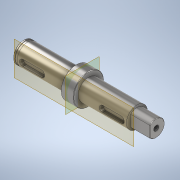
# Autodesk Inventor part: ParallelSystem_ProximalPart_Shaft_Driven_Rillenkugellager
Saved by Autodesk Inventor 2022 (Build 260153000, 153)
## iProperties
Created: 2022-07-19
Part Number: ParallelSystem_ProximalPart_Shaft_Driven_Rillenkugellager
Material: Edelstahl
Document SubType Name: Modeling
Designer: alexw
Density: 8 g/cm^3
Appearance: Halbpoliert
Mass: 39.624 g
Surface Area: 24.2962 cm^2
Volume: 4.95301 cm^3
ParrallelMecha_DrivenLink_OuterWidth: 52,000 mm
Querstrebe_Length: 36,000 mm
Author: alexw
Autodesk Inventor part; units mm, degrees
ref_plane "YZ Plane" through (0, 0, 0) normal (1, 0, 0) x (0, 1, 0)
ref_plane "XZ Plane" through (0, 0, 0) normal (0, 1, 0) x (-1, 0, 0)
sketch "Skizze1" plane through (0, 0, 0) normal (0, 0, 1) x (1, 0, 0)
  line L0 (0, 0) -> (0, 5)
  line L1 (0, 5) -> (0.8, 5)
  line L2 (0.8, 5) -> (0.8, 4.8)
  line L3 (0.8, 4.8) -> (1.9, 4.8)
  line L4 (1.9, 4.8) -> (1.9, 5)
  line L5 (1.9, 5) -> (24.9, 5)
  line L6 (24.9, 5) -> (24.9, 7.25)
  line L7 (24.9, 7.25) -> (30.9, 7.25)
  line L8 (30.9, 7.25) -> (30.9, 5)
  line L9 (30.9, 5) -> (53.9, 5)
  line L10 (53.9, 5) -> (53.9, 4)
  line L11 (53.9, 4) -> (63.1, 4)
  line L12 (63.1, 4) -> (63.1, 0)
  line L13 (63.1, 0) -> (0, 0)
  line L14 (15.9, 5) -> (15.9, 0) construction
  line L15 (39.9, 5) -> (39.9, 0) construction
  line L16 (9.9, 5) -> (9.9, 0) construction
  line L17 (45.9, 5) -> (45.9, 0) construction
  line L18 (53.9, 5) -> (53.9, 0) construction
  dimension "d0" = 10
  dimension "d2" = 14.5
  dimension "d3" = 1.1
  dimension "d4" = 9.6
  dimension "d5" = 0.8
  dimension "d7" = 9
  dimension "d8" = 9
  dimension "d9" = 6
  dimension "d10" = 14
  dimension "d11" = 14
  dimension "ParrallelMecha_DrivenLink_OuterWidth" = 52
  dimension "d22" = 6
  dimension "d23" = 6
  dimension "Querstrebe_Length" = 36
  dimension "d25" = 9.2
  dimension "d26" = 8
  constraints: 38 end point, 14 perpendicular, 13 point on line, 1 vertical
  measures "d0" diameter of L5 L13
  measures "d2" diameter of L7 L13
  measures "d3" distance of L3.end L2.end
  measures "d4" diameter of L3 L13
  measures "d5" distance between parallel lines of L2 L0
  measures "d7" distance between parallel lines of L6 L14
  measures "d8" distance between parallel lines of L8 L15
  measures "d9" distance between parallel lines of L8 L6
  measures "d10" distance between parallel lines of L4 L14
  measures "d11" distance between parallel lines of L15 L10
  measures "ParrallelMecha_DrivenLink_OuterWidth" distance between parallel lines of L10 L4
  measures "d22" distance between parallel lines of L15 L17
  measures "d23" distance between parallel lines of L16 L14
  measures "Querstrebe_Length" distance between parallel lines of L17 L16
  measures "d25" distance between parallel lines of L12 L18
  measures "d26" diameter of L11 L13
revolve "Umdrehung1" add sketch "Skizze1" angle 360 about axis through (63.1, 0, 0) along (-1, 0, 0)
chamfer "Fase1" distance 0.2 angle 45 4 edges at (24.9, -7.25, 0) (30.9, -7.25, 0) (63.1, -4, 0) (0, -5, 0)
ref_plane "Wellennut_Spiegelebene" through (27.9, 0, 0) normal (-1, 0, 0) x (0, 0, 1)
ref_plane "Arbeitsebene2" through (13.4, 0, 5) normal (0, 0, 1) x (1, 0, 0)
sketch "Skizze3" plane through (13.4, 0, 5) normal (0, 0, 1) x (1, 0, 0)
  line L0 (2.5, 5) -> (2.5, 0) construction
  line L1 (-26.02, 0) -> (62.32, 0) construction
  line L2 (0, 0) -> (-9, 0) construction
  line L3 (0, 1.5) -> (-9, 1.5)
  line L4 (-9, -1.5) -> (0, -1.5)
  arc A0 (0, -1.5) -> (0, 1.5) centre (0, 0) ccw
  arc A1 (-9, 1.5) -> (-9, -1.5) centre (-9, 0) ccw
  line L5 (-11.5, 0) -> (2.5, 0) construction
  line L6 (-11.5, -5) -> (-11.5, 5) construction
  point P0 (-13.4, 0)
  point P1 (-4.5, 0)
  point P2 (-4.5, 0)
  dimension "d17" = 3
  dimension "d18" = 12
  constraints: 10 end point, 4 point on circle, 4 tangent, 3 midpoint, 2 centre point, 2 horizontal, 2 point on line, 1 coincident, 1 collinear, 1 parallel
  measures "d17" distance between parallel lines of L4 L3
extrude "Wellennut" cut sketch "Skizze3" against normal blind 1.8
mirror "Spiegeln1" about plane through (27.9, 0, 0) normal (-1, 0, 0) of "Wellennut"
sketch "Skizze4" plane through (53.9, 0, 0) normal (1, 0, 0) x (0, 0, -1)
  circle A0 centre (0, 0) radius 4 projected
  line L0 (-3, -2.6458) -> (-3, 2.6458)
  point P0 (0, 0)
  dimension "d27" = 3
  constraints: 2 end point, 2 point on circle, 1 vertical
  measures "d27" distance from line of L0 point (0, 0)
extrude "Extrusion2" cut sketch "Skizze4" along normal through all contours L0 A0 picked at (-3.1815, -0.6179)
chamfer "Fase2" distance 0.2 angle 45 1 edges at (63.1, 0, 3)
sketch "Skizze5" plane through (63.1, 0, 0) normal (1, 0, 0) x (0, 0, -1)
  arc A0 (-3, -2.6458) -> (-3, 2.6458) centre (0, 0) ccw construction
  circle A1 centre (0, 0) radius 5 construction
  point P0 (0, 0)
  constraints: 1 coincident
hole "Bohrung1" at (63.1, 0, 0) direction (-1, 0, 0) diameter 2.459 depth 8 tip angle 118 thread size "M3x0.5" class "6H" standard "ISO Metric profile"
equation "\"d10\" = ParallelLink_Lever_Thickness + ParallelMecha_Bearing_Step_Thickness"
equation "\"d11\" = d10"
equation "\"d22\" = ParallelMecha_Bearing_Step_Thickness"
equation "\"d23\" = d22"
equation "\"d26\" = CapstonV2_ShaftDia"
equation "\"d27\" = 0.5 * CapstonV2_ShaftDia - Poligonprofil_Ausnehmung"
equation "\"ParallelLink_Lever_Thickness\" = 8"
equation "\"ParallelMecha_Bearing_Step_Thickness\" = 6"
equation "\"CapstonV2_ShaftDia\" = 8"
equation "\"Poligonprofil_Ausnehmung\" = 1"
